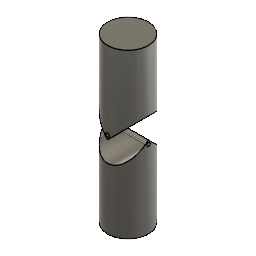
_double hinge.c73257d0-b62e-4581-b0a2-3ff71a05638e (Autodesk Fusion 360 design; units mm, degrees)
Autodesk Fusion 360 part; units mm, degrees
note: some values were not read from the file. Chosen so that the rebuilt part matches the saved one: which face or edge a step refers to.
sketch "Sketch1" plane through (0, 0, 0) normal (0, 1, 0) x (1, 0, 0)
  circle A0 centre (0, 0) radius 50
  dimension "d7" = 100
  measures "d7" diameter of A0
extrude "Extrude2" add sketch "Sketch1" along normal blind 300 makes body 1
sketch "Sketch2" plane through (0, 0, 0) normal (0, 0, 1) x (1, 0, 0)
sketch "Sketch3" plane through (0, 0, 0) normal (1, 0, 0) x (0, 0, -1)
  circle A0 centre (0, 0) radius 50
  dimension "d12" = 100
  measures "d12" diameter of A0
extrude "Extrude3" cut sketch "Sketch3" along normal through all and the other way through all bodies 1
sketch "Sketch4" plane through (0, 0, 0) normal (0, 1, 0) x (1, 0, 0)
sphere "SpherePrimitive1" add diameter 90 placed x (1, 0, 0) y (0, 0, -1) z (0, 1, 0) at (0, 0, 0) separate body makes body 2
pattern_circular "C-Pattern1" count 2 over 180 about axis through (1.75, 0, 0) along (1, 0, 0) of bodies 1 makes body 3
move_body "Move1" bodies 3 to x (0, 0, -1) y (0, 1, 0) z (1, 0, 0) at (0, 0, 0)
extrude "Extrude4" cut 1 faces at (-13.5518, 300, 2.484) along direction (0, -1, 0) blind 100 on bodies 1 bodies 1
extrude "Extrude5" cut 1 faces at (-2.484, -300, 13.5518) along direction (0, 1, 0) blind 100 on bodies 3 bodies 3
copy_body "Body->Comp1" bodies 3 removing the originals makes body 4 in component "Component"
copy_body "Body->Comp2" bodies 1 removing the originals makes body 5 in component "Component'"
copy_body "Body->Comp3" bodies 2 removing the originals makes body 6 in component "Component''"
sketch "Sketch5" plane through (0, 0, 0) normal (0, 0, 1) x (1, 0, 0)
  circle A0 centre (0, 0) radius 4.5
  dimension "d23" = 9
  measures "d23" diameter of A0
extrude "Extrude6" add sketch "Sketch5" along normal mid plane 100 separate body makes body 7
copy_body "Body->Comp4" bodies 7 removing the originals makes body 8 in component "Component'''"
move_face "MoveFace1" to x (1, 0, 0) y (0, 1, 0) z (0, 0, 1) at (0, 0, 170) 1 faces at (4.4776, -0.4481, 16.6667) on bodies 8 in component "Component'''"
sketch "Sketch6" plane through (0, 0, 0) normal (1, 0, 0) x (0, 0, -1)
  circle A0 centre (0, 0) radius 4.5
  dimension "d29" = 9
  measures "d29" diameter of A0
extrude "Extrude7" add sketch "Sketch6" along normal mid plane 100 separate body makes body 9
copy_body "Body->Comp5" bodies 9 removing the originals makes body 10 in component "Component''''"
move_body "MoveFace1'" bodies 10 to x (1, 0, 0) y (0, 1, 0) z (0, 0, 1) at (0, -10, 0) on bodies 10 in component "Component''''"
component "Component" placed x (1, 0, 0) y (0, 1, 0) z (0, 0, 1) at (0, 0, 0)
component "Component'" placed x (1, 0, 0) y (0, 1, 0) z (0, 0, 1) at (0, 0, 0)
component "Component''" placed x (1, 0, 0) y (0, 1, 0) z (0, 0, 1) at (0, 0, 0)
component "Component'''" placed x (1, 0, 0) y (0, 1, 0) z (0, 0, 1) at (0, 10, 0)
component "Component''''" placed x (1, 0, 0) y (0, 1, 0) z (0, 0, 1) at (0, 0, 0)
